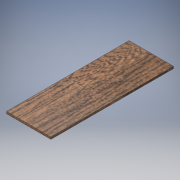
# Autodesk Inventor part: etage
Saved by Autodesk Inventor 2019 (Build 230136000, 136)
## iProperties
Created: 2020-02-16
Part Number: etage
Material: Generic
Document SubType Name: Modeling
Designer: franc
Density: 1 g/cm^3
Appearance: Default
Author: franc
Autodesk Inventor part; units mm, degrees
ref_plane "YZ Plane" through (0, 0, 0) normal (1, 0, 0) x (0, 1, 0)
ref_plane "XZ Plane" through (0, 0, 0) normal (0, 1, 0) x (-1, 0, 0)
ref_plane "XY Plane" through (0, 0, 0) normal (0, 0, 1) x (1, 0, 0)
sketch "Esquisse1" plane through (0, 0, 0) normal (0, 1, 0) x (-1, 0, 0)
  line L0 (51.7905, 152.7196) -> (-53.2095, 152.7196)
  line L1 (-53.2095, 152.7196) -> (-53.2095, -137.2804)
  line L2 (-53.2095, -137.2804) -> (51.7905, -137.2804)
  line L3 (51.7905, -137.2804) -> (51.7905, 152.7196)
  point P0 (0, 0)
  dimension "d0" = 105
  dimension "d1" = 290
  constraints: 8 end point, 2 parallel, 1 horizontal, 1 perpendicular
  measures "d0" distance of L1.end L2.end
  measures "d1" distance of L2.end L0.start
extrude "Extrusion1" add sketch "Esquisse1" along normal blind 5
